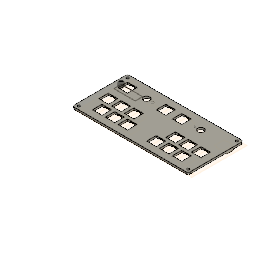
Keyboard Plate (Autodesk Fusion 360 design; units mm, degrees)
Autodesk Fusion 360 part; units mm, degrees
(part 1 of 2)
sketch "fe59f99c189e2fed6147eb83aa4c487c15dc8bc6_switch" plane through (0, 0, 0) normal (0, 0, 1) x (1, 0, 0)
  line L0 (34.1437, 24.5994) -> (34.1437, 10.5999)
  line L1 (110.63, 43.6492) -> (124.631, 43.6492)
  line L2 (58.2429, 24.5994) -> (72.2422, 24.5994)
  line L3 (110.63, 29.6499) -> (110.63, 43.6492)
  line L4 (29.6692, 43.6492) -> (43.6686, 43.6492)
  line L5 (43.6686, 29.6499) -> (29.6692, 29.6499)
  line L6 (124.631, 29.6499) -> (110.63, 29.6499)
  line L7 (101.105, 10.5999) -> (101.105, 24.5994)
  line L8 (120.155, 24.5994) -> (134.156, 24.5994)
  line L9 (53.1922, 24.5994) -> (53.1922, 10.5999)
  line L10 (129.68, 29.6499) -> (129.68, 43.6492)
  line L11 (67.7693, 72.2256) -> (81.7686, 72.2256)
  line L12 (148.73, 43.6492) -> (162.731, 43.6492)
  line L13 (115.106, 10.5999) -> (101.105, 10.5999)
  line L14 (20.1428, 10.5999) -> (20.1428, 24.5994)
  line L15 (148.73, 29.6499) -> (148.73, 43.6492)
  line L16 (34.1437, 10.5999) -> (20.1428, 10.5999)
  line L17 (62.7186, 43.6492) -> (62.7186, 29.6499)
  line L18 (24.6187, 29.6499) -> (10.6178, 29.6499)
  line L19 (120.155, 10.5999) -> (120.155, 24.5994)
  line L20 (134.156, 24.5994) -> (134.156, 10.5999)
  line L21 (153.206, 10.5999) -> (139.205, 10.5999)
  line L22 (10.6178, 43.6492) -> (24.6187, 43.6492)
  line L23 (143.681, 43.6492) -> (143.681, 29.6499)
  line L24 (139.205, 24.5994) -> (153.206, 24.5994)
  line L25 (20.1428, 24.5994) -> (34.1437, 24.5994)
  line L26 (39.1929, 10.5999) -> (39.1929, 24.5994)
  line L27 (162.731, 29.6499) -> (148.73, 29.6499)
  line L28 (124.631, 43.6492) -> (124.631, 29.6499)
  line L29 (58.2429, 10.5999) -> (58.2429, 24.5994)
  line L30 (134.156, 10.5999) -> (120.155, 10.5999)
  line L31 (48.7193, 43.6492) -> (62.7186, 43.6492)
  line L32 (153.206, 24.5994) -> (153.206, 10.5999)
  line L33 (143.681, 29.6499) -> (129.68, 29.6499)
  line L34 (162.731, 58.2249) -> (148.73, 58.2249)
  line L35 (115.106, 24.5994) -> (115.106, 10.5999)
  line L36 (0.0937, 82.7497) -> (173.257, 82.7497)
  line L37 (53.1922, 10.5999) -> (39.1929, 10.5999)
  line L38 (10.6178, 29.6499) -> (10.6178, 43.6492)
  line L39 (43.6686, 43.6492) -> (43.6686, 29.6499)
  line L40 (105.581, 58.2249) -> (91.5804, 58.2249)
  line L41 (67.7693, 58.2249) -> (67.7693, 72.2256)
  line L42 (62.7186, 29.6499) -> (48.7193, 29.6499)
  line L43 (81.7686, 58.2249) -> (67.7693, 58.2249)
  line L44 (148.73, 72.2256) -> (162.731, 72.2256)
  line L45 (0.0937, 0.0744) -> (0.0937, 82.7497)
  line L46 (173.257, 0.0744) -> (0.0937, 0.0744)
  line L47 (72.2422, 10.5999) -> (58.2429, 10.5999)
  line L48 (39.1929, 24.5994) -> (53.1922, 24.5994)
  line L49 (173.257, 82.7497) -> (173.257, 0.0744)
  line L50 (72.2422, 24.5994) -> (72.2422, 10.5999)
  line L51 (29.6692, 29.6499) -> (29.6692, 43.6492)
  line L52 (148.73, 58.2249) -> (148.73, 72.2256)
  line L53 (162.731, 43.6492) -> (162.731, 29.6499)
  line L54 (91.5804, 72.2256) -> (105.581, 72.2256)
  line L55 (139.205, 10.5999) -> (139.205, 24.5994)
  line L56 (91.5804, 58.2249) -> (91.5804, 72.2256)
  line L57 (81.7686, 72.2256) -> (81.7686, 58.2249)
  line L58 (24.6187, 43.6492) -> (24.6187, 29.6499)
  line L59 (48.7193, 29.6499) -> (48.7193, 43.6492)
  line L60 (129.68, 43.6492) -> (143.681, 43.6492)
  line L61 (162.731, 72.2256) -> (162.731, 58.2249)
  line L62 (105.581, 72.2256) -> (105.581, 58.2249)
  line L63 (101.105, 24.5994) -> (115.106, 24.5994)
extrude "Extrude1" add sketch "fe59f99c189e2fed6147eb83aa4c487c15dc8bc6_switch" along normal blind 3
sketch "Sketch2" plane through (0, 0, 3) normal (0, 0, 1) x (-1, 0, 0)
  line L0 (-39.1929, -10.5999) -> (-39.1929, -24.5994)
  line L1 (-39.1929, -24.5994) -> (-53.1922, -24.5994)
  line L2 (-53.1922, -24.5994) -> (-53.1922, -10.5999)
  line L3 (-53.1922, -10.5999) -> (-39.1929, -10.5999)
  line L4 (-110.63, -43.6492) -> (-124.631, -43.6492)
  line L5 (-124.631, -43.6492) -> (-124.631, -29.6499)
  line L6 (-124.631, -29.6499) -> (-110.63, -29.6499)
  line L7 (-110.63, -29.6499) -> (-110.63, -43.6492)
  line L8 (-134.156, -24.5994) -> (-134.156, -10.5999)
  line L9 (-134.156, -10.5999) -> (-120.155, -10.5999)
  line L10 (-120.155, -10.5999) -> (-120.155, -24.5994)
  line L11 (-120.155, -24.5994) -> (-134.156, -24.5994)
  line L12 (-20.1428, -10.5999) -> (-20.1428, -24.5994)
  line L13 (-20.1428, -24.5994) -> (-34.1437, -24.5994)
  line L14 (-34.1437, -24.5994) -> (-34.1437, -10.5999)
  line L15 (-34.1437, -10.5999) -> (-20.1428, -10.5999)
  line L16 (-148.73, -43.6492) -> (-162.731, -43.6492)
  line L17 (-162.731, -43.6492) -> (-162.731, -29.6499)
  line L18 (-162.731, -29.6499) -> (-148.73, -29.6499)
  line L19 (-148.73, -29.6499) -> (-148.73, -43.6492)
  line L20 (-58.2429, -24.5994) -> (-72.2422, -24.5994)
  line L21 (-72.2422, -24.5994) -> (-72.2422, -10.5999)
  line L22 (-72.2422, -10.5999) -> (-58.2429, -10.5999)
  line L23 (-58.2429, -10.5999) -> (-58.2429, -24.5994)
  line L24 (-43.6686, -29.6499) -> (-29.6692, -29.6499)
  line L25 (-29.6692, -29.6499) -> (-29.6692, -43.6492)
  line L26 (-29.6692, -43.6492) -> (-43.6686, -43.6492)
  line L27 (-43.6686, -43.6492) -> (-43.6686, -29.6499)
  line L28 (-153.206, -10.5999) -> (-139.205, -10.5999)
  line L29 (-139.205, -10.5999) -> (-139.205, -24.5994)
  line L30 (-139.205, -24.5994) -> (-153.206, -24.5994)
  line L31 (-153.206, -24.5994) -> (-153.206, -10.5999)
  line L32 (-10.6178, -43.6492) -> (-24.6187, -43.6492)
  line L33 (-24.6187, -43.6492) -> (-24.6187, -29.6499)
  line L34 (-24.6187, -29.6499) -> (-10.6178, -29.6499)
  line L35 (-10.6178, -29.6499) -> (-10.6178, -43.6492)
  line L36 (-62.7186, -29.6499) -> (-48.7193, -29.6499)
  line L37 (-48.7193, -29.6499) -> (-48.7193, -43.6492)
  line L38 (-48.7193, -43.6492) -> (-62.7186, -43.6492)
  line L39 (-62.7186, -43.6492) -> (-62.7186, -29.6499)
  line L40 (-67.7693, -72.2256) -> (-81.7686, -72.2256)
  line L41 (-81.7686, -72.2256) -> (-81.7686, -58.2249)
  line L42 (-81.7686, -58.2249) -> (-67.7693, -58.2249)
  line L43 (-67.7693, -58.2249) -> (-67.7693, -72.2256)
  line L44 (-129.68, -29.6499) -> (-129.68, -43.6492)
  line L45 (-129.68, -43.6492) -> (-143.681, -43.6492)
  line L46 (-143.681, -43.6492) -> (-143.681, -29.6499)
  line L47 (-143.681, -29.6499) -> (-129.68, -29.6499)
  line L48 (-148.73, -72.2256) -> (-162.731, -72.2256)
  line L49 (-162.731, -72.2256) -> (-162.731, -58.2249)
  line L50 (-162.731, -58.2249) -> (-148.73, -58.2249)
  line L51 (-148.73, -58.2249) -> (-148.73, -72.2256)
  line L52 (-101.105, -10.5999) -> (-101.105, -24.5994)
  line L53 (-101.105, -24.5994) -> (-115.106, -24.5994)
  line L54 (-115.106, -24.5994) -> (-115.106, -10.5999)
  line L55 (-115.106, -10.5999) -> (-101.105, -10.5999)
  line L56 (-91.5804, -72.2256) -> (-105.581, -72.2256)
  line L57 (-105.581, -72.2256) -> (-105.581, -58.2249)
  line L58 (-105.581, -58.2249) -> (-91.5804, -58.2249)
  line L59 (-91.5804, -58.2249) -> (-91.5804, -72.2256)
  line L60 (-173.257, -82.7497) -> (-0.0937, -82.7497)
  line L61 (-0.0937, -82.7497) -> (-0.0937, -0.0744)
  line L62 (-0.0937, -0.0744) -> (-173.257, -0.0744)
  line L63 (-173.257, -0.0744) -> (-173.257, -82.7497)
  line L64 (-71.769, -72.2256) -> (-77.769, -72.2256)
  line L65 (-77.769, -72.2256) -> (-77.769, -73.2256)
  line L66 (-77.769, -73.2256) -> (-71.769, -73.2256)
  line L67 (-71.769, -73.2256) -> (-71.769, -72.2256)
  line L68 (-71.769, -58.2249) -> (-77.769, -58.2249)
  line L69 (-77.769, -58.2249) -> (-77.769, -57.2249)
  line L70 (-77.769, -57.2249) -> (-71.769, -57.2249)
  line L71 (-71.769, -57.2249) -> (-71.769, -58.2249)
  line L72 (-95.5807, -58.2249) -> (-101.5807, -58.2249)
  line L73 (-101.5807, -73.2256) -> (-95.5807, -73.2256)
  line L74 (-101.5807, -72.2256) -> (-101.5807, -73.2256)
  line L75 (-95.5807, -72.2256) -> (-101.5807, -72.2256)
  line L76 (-95.5807, -73.2256) -> (-95.5807, -72.2256)
  line L77 (-101.5807, -58.2249) -> (-101.5807, -57.2249)
  line L78 (-95.5807, -57.2249) -> (-95.5807, -58.2249)
  line L79 (-101.5807, -57.2249) -> (-95.5807, -57.2249)
  line L80 (-152.7305, -58.2249) -> (-158.7305, -58.2249)
  line L81 (-158.7305, -73.2256) -> (-152.7305, -73.2256)
  line L82 (-158.7305, -72.2256) -> (-158.7305, -73.2256)
  line L83 (-152.7305, -72.2256) -> (-158.7305, -72.2256)
  line L84 (-152.7305, -73.2256) -> (-152.7305, -72.2256)
  line L85 (-158.7305, -58.2249) -> (-158.7305, -57.2249)
  line L86 (-152.7305, -57.2249) -> (-152.7305, -58.2249)
  line L87 (-158.7305, -57.2249) -> (-152.7305, -57.2249)
  line L88 (-14.6183, -43.6492) -> (-20.6183, -43.6492)
  line L89 (-20.6183, -43.6492) -> (-20.6183, -44.6492)
  line L90 (-20.6183, -44.6492) -> (-14.6183, -44.6492)
  line L91 (-14.6183, -44.6492) -> (-14.6183, -43.6492)
  line L92 (-14.6183, -29.6499) -> (-20.6183, -29.6499)
  line L93 (-20.6183, -29.6499) -> (-20.6183, -28.6499)
  line L94 (-20.6183, -28.6499) -> (-14.6183, -28.6499)
  line L95 (-14.6183, -28.6499) -> (-14.6183, -29.6499)
  line L96 (-58.719, -29.6499) -> (-58.719, -28.6499)
  line L97 (-58.719, -28.6499) -> (-52.7189, -28.6499)
  line L98 (-58.7189, -44.6492) -> (-52.7189, -44.6492)
  line L99 (-52.7189, -29.6499) -> (-58.719, -29.6499)
  line L100 (-52.7189, -43.6492) -> (-58.7189, -43.6492)
  line L101 (-52.7189, -44.6492) -> (-52.7189, -43.6492)
  line L102 (-58.7189, -43.6492) -> (-58.7189, -44.6492)
  line L103 (-52.7189, -28.6499) -> (-52.7189, -29.6499)
  line L104 (-39.6689, -29.6499) -> (-39.6689, -28.6499)
  line L105 (-39.6689, -28.6499) -> (-33.6689, -28.6499)
  line L106 (-39.6689, -44.6492) -> (-33.6689, -44.6492)
  line L107 (-33.6689, -29.6499) -> (-39.6689, -29.6499)
  line L108 (-33.6689, -43.6492) -> (-39.6689, -43.6492)
  line L109 (-33.6689, -44.6492) -> (-33.6689, -43.6492)
  line L110 (-39.6689, -43.6492) -> (-39.6689, -44.6492)
  line L111 (-33.6689, -28.6499) -> (-33.6689, -29.6499)
  line L112 (-120.6305, -29.6499) -> (-120.6305, -28.6499)
  line L113 (-120.6305, -28.6499) -> (-114.6305, -28.6499)
  line L114 (-120.6305, -44.6492) -> (-114.6305, -44.6492)
  line L115 (-114.6305, -29.6499) -> (-120.6305, -29.6499)
  line L116 (-114.6305, -43.6492) -> (-120.6305, -43.6492)
  line L117 (-114.6305, -44.6492) -> (-114.6305, -43.6492)
  line L118 (-120.6305, -43.6492) -> (-120.6305, -44.6492)
  line L119 (-114.6305, -28.6499) -> (-114.6305, -29.6499)
  line L120 (-139.6805, -29.6499) -> (-139.6805, -28.6499)
  line L121 (-139.6805, -28.6499) -> (-133.6805, -28.6499)
  line L122 (-139.6805, -44.6492) -> (-133.6805, -44.6492)
  line L123 (-133.6805, -29.6499) -> (-139.6805, -29.6499)
  line L124 (-133.6805, -43.6492) -> (-139.6805, -43.6492)
  line L125 (-133.6805, -44.6492) -> (-133.6805, -43.6492)
  line L126 (-139.6805, -43.6492) -> (-139.6805, -44.6492)
  line L127 (-133.6805, -28.6499) -> (-133.6805, -29.6499)
  line L128 (-158.7305, -29.6499) -> (-158.7305, -28.6499)
  line L129 (-158.7305, -28.6499) -> (-152.7305, -28.6499)
  line L130 (-158.7305, -44.6492) -> (-152.7305, -44.6492)
  line L131 (-152.7305, -29.6499) -> (-158.7305, -29.6499)
  line L132 (-152.7305, -43.6492) -> (-158.7305, -43.6492)
  line L133 (-152.7305, -44.6492) -> (-152.7305, -43.6492)
  line L134 (-158.7305, -43.6492) -> (-158.7305, -44.6492)
  line L135 (-152.7305, -28.6499) -> (-152.7305, -29.6499)
  line L136 (-24.1433, -24.5994) -> (-30.1433, -24.5994)
  line L137 (-30.1433, -24.5994) -> (-30.1433, -25.5994)
  line L138 (-30.1433, -25.5994) -> (-24.1433, -25.5994)
  line L139 (-24.1433, -25.5994) -> (-24.1433, -24.5994)
  line L140 (-24.1433, -10.5999) -> (-30.1433, -10.5999)
  line L141 (-30.1433, -10.5999) -> (-30.1433, -9.5999)
  line L142 (-30.1433, -9.5999) -> (-24.1433, -9.5999)
  line L143 (-24.1433, -9.5999) -> (-24.1433, -10.5999)
  line L144 (-43.1926, -9.5999) -> (-43.1926, -10.5999)
  line L145 (-49.1926, -9.5999) -> (-43.1926, -9.5999)
  line L146 (-49.1926, -24.5994) -> (-49.1926, -25.5994)
  line L147 (-43.1926, -10.5999) -> (-49.1926, -10.5999)
  line L148 (-43.1926, -24.5994) -> (-49.1926, -24.5994)
  line L149 (-43.1926, -25.5994) -> (-43.1926, -24.5994)
  line L150 (-49.1926, -10.5999) -> (-49.1926, -9.5999)
  line L151 (-49.1926, -25.5994) -> (-43.1926, -25.5994)
  line L152 (-62.2426, -9.5999) -> (-62.2426, -10.5999)
  line L153 (-68.2426, -9.5999) -> (-62.2426, -9.5999)
  line L154 (-68.2425, -24.5994) -> (-68.2425, -25.5994)
  line L155 (-62.2426, -10.5999) -> (-68.2426, -10.5999)
  line L156 (-62.2426, -24.5994) -> (-68.2425, -24.5994)
  line L157 (-62.2426, -25.5994) -> (-62.2426, -24.5994)
  line L158 (-68.2426, -10.5999) -> (-68.2426, -9.5999)
  line L159 (-68.2425, -25.5994) -> (-62.2425, -25.5994)
  line L160 (-105.1055, -9.5999) -> (-105.1055, -10.5999)
  line L161 (-111.1055, -9.5999) -> (-105.1055, -9.5999)
  line L162 (-111.1055, -24.5994) -> (-111.1055, -25.5994)
  line L163 (-105.1055, -10.5999) -> (-111.1055, -10.5999)
  line L164 (-105.1055, -24.5994) -> (-111.1055, -24.5994)
  line L165 (-105.1055, -25.5994) -> (-105.1055, -24.5994)
  line L166 (-111.1055, -10.5999) -> (-111.1055, -9.5999)
  line L167 (-111.1055, -25.5994) -> (-105.1055, -25.5994)
  line L168 (-124.1555, -9.5999) -> (-124.1555, -10.5999)
  line L169 (-130.1555, -9.5999) -> (-124.1555, -9.5999)
  line L170 (-130.1555, -24.5994) -> (-130.1555, -25.5994)
  line L171 (-124.1555, -10.5999) -> (-130.1555, -10.5999)
  line L172 (-124.1555, -24.5994) -> (-130.1555, -24.5994)
  line L173 (-124.1555, -25.5994) -> (-124.1555, -24.5994)
  line L174 (-130.1555, -10.5999) -> (-130.1555, -9.5999)
  line L175 (-130.1555, -25.5994) -> (-124.1555, -25.5994)
  line L176 (-143.2055, -9.5999) -> (-143.2055, -10.5999)
  line L177 (-149.2055, -9.5999) -> (-143.2055, -9.5999)
  line L178 (-149.2055, -24.5994) -> (-149.2055, -25.5994)
  line L179 (-143.2055, -10.5999) -> (-149.2055, -10.5999)
  line L180 (-143.2055, -24.5994) -> (-149.2055, -24.5994)
  line L181 (-143.2055, -25.5994) -> (-143.2055, -24.5994)
  line L182 (-149.2055, -10.5999) -> (-149.2055, -9.5999)
  line L183 (-149.2055, -25.5994) -> (-143.2055, -25.5994)
  dimension "d3" = 6
  dimension "d4" = 1
  dimension "d5" = 6
  dimension "d6" = 1
  dimension "d7" = 6
  dimension "d8" = 1
  dimension "d9" = 6
  dimension "d10" = 1
  dimension "d11" = 6
  dimension "d12" = 1
  dimension "d13" = 6
  dimension "d14" = 1
  dimension "d15" = 6
  dimension "d16" = 1
  dimension "d17" = 6
  dimension "d18" = 1
  dimension "d19" = 6
  dimension "d20" = 1
  dimension "d21" = 6
  dimension "d22" = 1
  dimension "d23" = 6
  dimension "d24" = 1
  dimension "d25" = 6
  dimension "d26" = 1
  dimension "d27" = 6
  dimension "d28" = 1
  dimension "d29" = 6
  dimension "d30" = 1
  dimension "d31" = 6
  dimension "d32" = 1
  dimension "d33" = 6
  dimension "d34" = 1
  dimension "d35" = 6
  dimension "d36" = 1
  dimension "d37" = 6
  dimension "d38" = 1
  dimension "d39" = 6
  dimension "d40" = 1
  dimension "d41" = 6
  dimension "d42" = 1
  dimension "d43" = 6
  dimension "d44" = 1
  dimension "d45" = 6
  dimension "d46" = 1
  dimension "d47" = 6
  dimension "d48" = 1
  dimension "d49" = 6
  dimension "d50" = 1
  dimension "d51" = 6
  dimension "d52" = 1
  dimension "d53" = 6
  dimension "d54" = 1
  dimension "d55" = 6
  dimension "d56" = 1
  dimension "d57" = 6
  dimension "d58" = 1
  dimension "d59" = 6
  dimension "d60" = 1
  dimension "d61" = 6
  dimension "d62" = 1
  constraint horizontal L64
  constraint vertical L65
  constraint horizontal L66
  constraint vertical L67
  constraint coincident L40 L64.start
  constraint horizontal L68
  constraint vertical L69
  constraint horizontal L70
  constraint vertical L71
  constraint coincident L42 L68.start
  constraint horizontal L75
  constraint vertical L74
  constraint horizontal L73
  constraint vertical L76
  constraint horizontal L72
  constraint vertical L77
  constraint horizontal L79
  constraint vertical L78
  constraint horizontal L83
  constraint vertical L82
  constraint horizontal L81
  constraint vertical L84
  constraint horizontal L80
  constraint vertical L85
  constraint horizontal L87
  constraint vertical L86
  constraint horizontal L88
  constraint vertical L89
  constraint horizontal L90
  constraint vertical L91
  constraint coincident L32 L88.start
  constraint horizontal L92
  constraint vertical L93
  constraint horizontal L94
  constraint vertical L95
  constraint coincident L34 L92.start
  constraint horizontal L100
  constraint vertical L102
  constraint horizontal L98
  constraint vertical L101
  constraint horizontal L99
  constraint vertical L96
  constraint horizontal L97
  constraint vertical L103
  constraint horizontal L108
  constraint vertical L110
  constraint horizontal L106
  constraint vertical L109
  constraint horizontal L107
  constraint vertical L104
  constraint horizontal L105
  constraint vertical L111
  constraint horizontal L116
  constraint vertical L118
  constraint horizontal L114
  constraint vertical L117
  constraint horizontal L115
  constraint vertical L112
  constraint horizontal L113
  constraint vertical L119
  constraint horizontal L124
  constraint vertical L126
  constraint horizontal L122
  constraint vertical L125
  constraint horizontal L123
  constraint vertical L120
  constraint horizontal L121
  constraint vertical L127
  constraint horizontal L132
  constraint vertical L134
  constraint horizontal L130
  constraint vertical L133
  constraint horizontal L131
  constraint vertical L128
  constraint horizontal L129
  constraint vertical L135
  constraint horizontal L136
  constraint vertical L137
  constraint horizontal L138
  constraint vertical L139
  constraint coincident L13 L136.start
  constraint horizontal L140
  constraint vertical L141
  constraint horizontal L142
  constraint vertical L143
  constraint coincident L15 L140.start
  constraint horizontal L148
  constraint vertical L146
  constraint horizontal L151
  constraint vertical L149
  constraint horizontal L147
  constraint vertical L150
  constraint horizontal L145
  constraint vertical L144
  constraint horizontal L156
  constraint vertical L154
  constraint horizontal L159
  constraint vertical L157
  constraint horizontal L155
  constraint vertical L158
  constraint horizontal L153
  constraint vertical L152
  constraint horizontal L164
  constraint vertical L162
  constraint horizontal L167
  constraint vertical L165
  constraint horizontal L163
  constraint vertical L166
  constraint horizontal L161
  constraint vertical L160
  constraint horizontal L172
  constraint vertical L170
  constraint horizontal L175
  constraint vertical L173
  constraint horizontal L171
  constraint vertical L174
  constraint horizontal L169
  constraint vertical L168
  constraint horizontal L180
  constraint vertical L178
  constraint horizontal L183
  constraint vertical L181
  constraint horizontal L179
  constraint vertical L182
  constraint horizontal L177
  constraint vertical L176
  constraint midpoint L40 L64
  constraint midpoint L56 L75
  constraint midpoint L58 L72
  constraint midpoint L42 L68
  constraint midpoint L48 L83
  constraint midpoint L50 L80
  constraint midpoint L16 L132
  constraint midpoint L45 L124
  constraint midpoint L18 L131
  constraint midpoint L47 L123
  constraint midpoint L6 L115
  constraint midpoint L4 L116
  constraint midpoint L38 L100
  constraint midpoint L36 L99
  constraint midpoint L24 L107
  constraint midpoint L26 L108
  constraint midpoint L32 L88
  constraint midpoint L34 L92
  constraint midpoint L13 L136
  constraint midpoint L15 L140
  constraint midpoint L3 L147
  constraint midpoint L1 L148
  constraint midpoint L20 L156
  constraint midpoint L22 L155
  constraint midpoint L55 L163
  constraint midpoint L53 L164
  constraint midpoint L11 L172
  constraint midpoint L9 L171
  constraint midpoint L28 L179
  constraint midpoint L30 L180
  measures "d3" distance of L64.start L64.end
  measures "d4" distance of L64.start L66.end
  measures "d5" distance of L68.start L68.end
  measures "d6" distance of L68.start L70.end
  measures "d7" distance of L75.start L74.start
  measures "d8" distance of L75.start L73.end
  measures "d9" distance of L72.start L72.end
  measures "d10" distance of L72.start L78.start
  measures "d11" distance of L83.start L82.start
  measures "d12" distance of L83.start L81.end
  measures "d13" distance of L80.start L80.end
  measures "d14" distance of L80.start L86.start
  measures "d15" distance of L88.start L88.end
  measures "d16" distance of L88.start L90.end
  measures "d17" distance of L92.start L92.end
  measures "d18" distance of L92.start L94.end
  measures "d19" distance of L100.end L100.start
  measures "d20" distance of L100.start L98.end
  measures "d21" distance of L96.start L99.start
  measures "d22" distance of L97.end L99.start
  measures "d23" distance of L108.end L108.start
  measures "d24" distance of L108.start L106.end
  measures "d25" distance of L104.start L107.start
  measures "d26" distance of L105.end L107.start
  measures "d27" distance of L116.end L116.start
  measures "d28" distance of L116.start L114.end
  measures "d29" distance of L112.start L115.start
  measures "d30" distance of L113.end L115.start
  measures "d31" distance of L124.end L124.start
  measures "d32" distance of L124.start L122.end
  measures "d33" distance of L120.start L123.start
  measures "d34" distance of L121.end L123.start
  measures "d35" distance of L132.end L132.start
  measures "d36" distance of L132.start L130.end
  measures "d37" distance of L128.start L131.start
  measures "d38" distance of L129.end L131.start
  measures "d39" distance of L136.start L136.end
  measures "d40" distance of L136.start L138.end
  measures "d41" distance of L140.start L140.end
  measures "d42" distance of L140.start L142.end
  measures "d43" distance of L148.start L146.start
  measures "d44" distance of L149.start L148.start
  measures "d45" distance of L144.end L147.end
  measures "d46" distance of L144.start L144.end
  measures "d47" distance of L156.start L154.start
  measures "d48" distance of L157.start L156.start
  measures "d49" distance of L152.end L155.end
  measures "d50" distance of L152.start L152.end
  measures "d51" distance of L164.start L162.start
  measures "d52" distance of L165.start L164.start
  measures "d53" distance of L160.end L163.end
  measures "d54" distance of L160.start L160.end
  measures "d55" distance of L172.start L170.start
  measures "d56" distance of L173.start L172.start
  measures "d57" distance of L168.end L171.end
  measures "d58" distance of L168.start L168.end
  measures "d59" distance of L180.start L178.start
  measures "d60" distance of L181.start L180.start
  measures "d61" distance of L176.end L179.end
  measures "d62" distance of L176.start L176.end
extrude "Extrude2" cut sketch "Sketch2" against normal blind 1.5 contours L3 L144 L145 L147 L150 | L1 L146 L148 L149 L151 | L4 L114 L116 L117 L118 | L6 L112 L113 L115 L119 | L11 L170 L172 L173 L175 | L9 L168 L169 L171 L174 | L15 L140 L141 L142 L143 | L13 L136 L137 L138 L139 | L16 L130 L132 L133 L134 | L18 L128 L129 L131 L135 | L20 L154 L156 L157 L159 | L22 L152 L153 L155 L158 | L24 L104 L105 L107 L111 | L26 L106 L108 L109 L110 | L28 L176 L177 L179 L182 | L30 L178 L180 L181 L183 | L32 L88 L89 L90 L91 | L34 L92 L93 L94 L95 | L36 L96 L97 L99 L103 | L38 L98 L100 L101 L102 | L40 L64 L65 L66 L67 | L42 L68 L69 L70 L71 | L47 L120 L121 L123 L127 | L45 L122 L124 L125 L126 | L48 L81 L82 L83 L84 | L50 L80 L85 L86 L87 | L55 L160 L161 L163 L166 | L53 L162 L164 L165 L167 | L56 L73 L74 L75 L76 | L58 L72 L77 L78 L79
sketch "Sketch3" plane through (0, 0, 3) normal (0, 0, 1) x (-1, 0, 0)
  line L0 (-173.257, -82.7497) -> (-0.0937, -82.7497)
  line L1 (-0.0937, -82.7497) -> (-0.0937, -0.0744)
  line L2 (-0.0937, -0.0744) -> (-173.257, -0.0744)
  line L3 (-173.257, -0.0744) -> (-173.257, -82.7497)
  line L4 (-101.5807, -58.2249) -> (-101.5807, -57.2249)
  line L5 (-101.5807, -57.2249) -> (-95.5807, -57.2249)
  line L6 (-95.5807, -57.2249) -> (-95.5807, -58.2249)
  line L7 (-95.5807, -58.2249) -> (-91.5804, -58.2249)
  line L8 (-91.5804, -58.2249) -> (-91.5804, -72.2256)
  line L9 (-91.5804, -72.2256) -> (-95.5807, -72.2256)
  line L10 (-95.5807, -72.2256) -> (-95.5807, -73.2256)
  line L11 (-95.5807, -73.2256) -> (-101.5807, -73.2256)
  line L12 (-101.5807, -73.2256) -> (-101.5807, -72.2256)
  line L13 (-101.5807, -72.2256) -> (-105.581, -72.2256)
  line L14 (-105.581, -72.2256) -> (-105.581, -58.2249)
  line L15 (-105.581, -58.2249) -> (-101.5807, -58.2249)
  line L16 (-152.7305, -72.2256) -> (-152.7305, -73.2256)
  line L17 (-152.7305, -73.2256) -> (-158.7305, -73.2256)
  line L18 (-158.7305, -73.2256) -> (-158.7305, -72.2256)
  line L19 (-158.7305, -72.2256) -> (-162.731, -72.2256)
  line L20 (-162.731, -72.2256) -> (-162.731, -58.2249)
  line L21 (-162.731, -58.2249) -> (-158.7305, -58.2249)
  line L22 (-158.7305, -58.2249) -> (-158.7305, -57.2249)
  line L23 (-158.7305, -57.2249) -> (-152.7305, -57.2249)
  line L24 (-152.7305, -57.2249) -> (-152.7305, -58.2249)
  line L25 (-152.7305, -58.2249) -> (-148.73, -58.2249)
  line L26 (-148.73, -58.2249) -> (-148.73, -72.2256)
  line L27 (-148.73, -72.2256) -> (-152.7305, -72.2256)
  line L28 (-58.7189, -44.6492) -> (-58.7189, -43.6492)
  line L29 (-58.7189, -43.6492) -> (-62.7186, -43.6492)
  line L30 (-62.7186, -43.6492) -> (-62.7186, -29.6499)
  line L31 (-62.7186, -29.6499) -> (-58.719, -29.6499)
  line L32 (-58.719, -29.6499) -> (-58.719, -28.6499)
  line L33 (-58.719, -28.6499) -> (-52.7189, -28.6499)
  line L34 (-52.7189, -28.6499) -> (-52.7189, -29.6499)
  line L35 (-52.7189, -29.6499) -> (-48.7193, -29.6499)
  line L36 (-48.7193, -29.6499) -> (-48.7193, -43.6492)
  line L37 (-48.7193, -43.6492) -> (-52.7189, -43.6492)
  line L38 (-52.7189, -43.6492) -> (-52.7189, -44.6492)
  line L39 (-52.7189, -44.6492) -> (-58.7189, -44.6492)
  line L40 (-24.1433, -24.5994) -> (-24.1433, -25.5994)
  line L41 (-24.1433, -25.5994) -> (-30.1433, -25.5994)
  line L42 (-30.1433, -25.5994) -> (-30.1433, -24.5994)
  line L43 (-30.1433, -24.5994) -> (-34.1437, -24.5994)
  line L44 (-34.1437, -24.5994) -> (-34.1437, -10.5999)
  line L45 (-34.1437, -10.5999) -> (-30.1433, -10.5999)
  line L46 (-30.1433, -10.5999) -> (-30.1433, -9.5999)
  line L47 (-30.1433, -9.5999) -> (-24.1433, -9.5999)
  line L48 (-24.1433, -9.5999) -> (-24.1433, -10.5999)
  line L49 (-24.1433, -10.5999) -> (-20.1428, -10.5999)
  line L50 (-20.1428, -10.5999) -> (-20.1428, -24.5994)
  line L51 (-20.1428, -24.5994) -> (-24.1433, -24.5994)
  line L52 (-71.769, -72.2256) -> (-71.769, -73.2256)
  line L53 (-71.769, -73.2256) -> (-77.769, -73.2256)
  line L54 (-77.769, -73.2256) -> (-77.769, -72.2256)
  line L55 (-77.769, -72.2256) -> (-81.7686, -72.2256)
  line L56 (-81.7686, -72.2256) -> (-81.7686, -58.2249)
  line L57 (-81.7686, -58.2249) -> (-77.769, -58.2249)
  line L58 (-77.769, -58.2249) -> (-77.769, -57.2249)
  line L59 (-77.769, -57.2249) -> (-71.769, -57.2249)
  line L60 (-71.769, -57.2249) -> (-71.769, -58.2249)
  line L61 (-71.769, -58.2249) -> (-67.7693, -58.2249)
  line L62 (-67.7693, -58.2249) -> (-67.7693, -72.2256)
  line L63 (-67.7693, -72.2256) -> (-71.769, -72.2256)
  line L64 (-158.7305, -44.6492) -> (-158.7305, -43.6492)
  line L65 (-158.7305, -43.6492) -> (-162.731, -43.6492)
  line L66 (-162.731, -43.6492) -> (-162.731, -29.6499)
  line L67 (-162.731, -29.6499) -> (-158.7305, -29.6499)
  line L68 (-158.7305, -29.6499) -> (-158.7305, -28.6499)
  line L69 (-158.7305, -28.6499) -> (-152.7305, -28.6499)
  line L70 (-152.7305, -28.6499) -> (-152.7305, -29.6499)
  line L71 (-152.7305, -29.6499) -> (-148.73, -29.6499)
  line L72 (-148.73, -29.6499) -> (-148.73, -43.6492)
  line L73 (-148.73, -43.6492) -> (-152.7305, -43.6492)
  line L74 (-152.7305, -43.6492) -> (-152.7305, -44.6492)
  line L75 (-152.7305, -44.6492) -> (-158.7305, -44.6492)
  line L76 (-149.2055, -25.5994) -> (-149.2055, -24.5994)
  line L77 (-149.2055, -24.5994) -> (-153.206, -24.5994)
  line L78 (-153.206, -24.5994) -> (-153.206, -10.5999)
  line L79 (-153.206, -10.5999) -> (-149.2055, -10.5999)
  line L80 (-149.2055, -10.5999) -> (-149.2055, -9.5999)
  line L81 (-149.2055, -9.5999) -> (-143.2055, -9.5999)
  line L82 (-143.2055, -9.5999) -> (-143.2055, -10.5999)
  line L83 (-143.2055, -10.5999) -> (-139.205, -10.5999)
  line L84 (-139.205, -10.5999) -> (-139.205, -24.5994)
  line L85 (-139.205, -24.5994) -> (-143.2055, -24.5994)
  line L86 (-143.2055, -24.5994) -> (-143.2055, -25.5994)
  line L87 (-143.2055, -25.5994) -> (-149.2055, -25.5994)
  line L88 (-62.2426, -9.5999) -> (-62.2426, -10.5999)
  line L89 (-62.2426, -10.5999) -> (-58.2429, -10.5999)
  line L90 (-58.2429, -10.5999) -> (-58.2429, -24.5994)
  line L91 (-58.2429, -24.5994) -> (-62.2426, -24.5994)
  line L92 (-62.2426, -24.5994) -> (-62.2426, -25.5994)
  line L93 (-62.2426, -25.5994) -> (-68.2425, -25.5994)
  line L94 (-68.2425, -25.5994) -> (-68.2425, -24.5994)
  line L95 (-68.2425, -24.5994) -> (-72.2422, -24.5994)
  line L96 (-72.2422, -24.5994) -> (-72.2422, -10.5999)
  line L97 (-72.2422, -10.5999) -> (-68.2426, -10.5999)
  line L98 (-68.2426, -10.5999) -> (-68.2426, -9.5999)
  line L99 (-68.2426, -9.5999) -> (-62.2426, -9.5999)
  line L100 (-114.6305, -28.6499) -> (-114.6305, -29.6499)
  line L101 (-114.6305, -29.6499) -> (-110.63, -29.6499)
  line L102 (-110.63, -29.6499) -> (-110.63, -43.6492)
  line L103 (-110.63, -43.6492) -> (-114.6305, -43.6492)
  line L104 (-114.6305, -43.6492) -> (-114.6305, -44.6492)
  line L105 (-114.6305, -44.6492) -> (-120.6305, -44.6492)
  line L106 (-120.6305, -44.6492) -> (-120.6305, -43.6492)
  line L107 (-120.6305, -43.6492) -> (-124.631, -43.6492)
  line L108 (-124.631, -43.6492) -> (-124.631, -29.6499)
  line L109 (-124.631, -29.6499) -> (-120.6305, -29.6499)
  line L110 (-120.6305, -29.6499) -> (-120.6305, -28.6499)
  line L111 (-120.6305, -28.6499) -> (-114.6305, -28.6499)
  line L112 (-111.1055, -25.5994) -> (-111.1055, -24.5994)
  line L113 (-111.1055, -24.5994) -> (-115.106, -24.5994)
  line L114 (-115.106, -24.5994) -> (-115.106, -10.5999)
  line L115 (-115.106, -10.5999) -> (-111.1055, -10.5999)
  line L116 (-111.1055, -10.5999) -> (-111.1055, -9.5999)
  line L117 (-111.1055, -9.5999) -> (-105.1055, -9.5999)
  line L118 (-105.1055, -9.5999) -> (-105.1055, -10.5999)
  line L119 (-105.1055, -10.5999) -> (-101.105, -10.5999)
  line L120 (-101.105, -10.5999) -> (-101.105, -24.5994)
  line L121 (-101.105, -24.5994) -> (-105.1055, -24.5994)
  line L122 (-105.1055, -24.5994) -> (-105.1055, -25.5994)
  line L123 (-105.1055, -25.5994) -> (-111.1055, -25.5994)
  line L124 (-14.6183, -43.6492) -> (-14.6183, -44.6492)
  line L125 (-14.6183, -44.6492) -> (-20.6183, -44.6492)
  line L126 (-20.6183, -44.6492) -> (-20.6183, -43.6492)
  line L127 (-20.6183, -43.6492) -> (-24.6187, -43.6492)
  line L128 (-24.6187, -43.6492) -> (-24.6187, -29.6499)
  line L129 (-24.6187, -29.6499) -> (-20.6183, -29.6499)
  line L130 (-20.6183, -29.6499) -> (-20.6183, -28.6499)
  line L131 (-20.6183, -28.6499) -> (-14.6183, -28.6499)
  line L132 (-14.6183, -28.6499) -> (-14.6183, -29.6499)
  line L133 (-14.6183, -29.6499) -> (-10.6178, -29.6499)
  line L134 (-10.6178, -29.6499) -> (-10.6178, -43.6492)
  line L135 (-10.6178, -43.6492) -> (-14.6183, -43.6492)
  line L136 (-130.1555, -25.5994) -> (-130.1555, -24.5994)
  line L137 (-130.1555, -24.5994) -> (-134.156, -24.5994)
  line L138 (-134.156, -24.5994) -> (-134.156, -10.5999)
  line L139 (-134.156, -10.5999) -> (-130.1555, -10.5999)
  line L140 (-130.1555, -10.5999) -> (-130.1555, -9.5999)
  line L141 (-130.1555, -9.5999) -> (-124.1555, -9.5999)
  line L142 (-124.1555, -9.5999) -> (-124.1555, -10.5999)
  line L143 (-124.1555, -10.5999) -> (-120.155, -10.5999)
  line L144 (-120.155, -10.5999) -> (-120.155, -24.5994)
  line L145 (-120.155, -24.5994) -> (-124.1555, -24.5994)
  line L146 (-124.1555, -24.5994) -> (-124.1555, -25.5994)
  line L147 (-124.1555, -25.5994) -> (-130.1555, -25.5994)
  line L148 (-133.6805, -28.6499) -> (-133.6805, -29.6499)
  line L149 (-133.6805, -29.6499) -> (-129.68, -29.6499)
  line L150 (-129.68, -29.6499) -> (-129.68, -43.6492)
  line L151 (-129.68, -43.6492) -> (-133.6805, -43.6492)
  line L152 (-133.6805, -43.6492) -> (-133.6805, -44.6492)
  line L153 (-133.6805, -44.6492) -> (-139.6805, -44.6492)
  line L154 (-139.6805, -44.6492) -> (-139.6805, -43.6492)
  line L155 (-139.6805, -43.6492) -> (-143.681, -43.6492)
  line L156 (-143.681, -43.6492) -> (-143.681, -29.6499)
  line L157 (-143.681, -29.6499) -> (-139.6805, -29.6499)
  line L158 (-139.6805, -29.6499) -> (-139.6805, -28.6499)
  line L159 (-139.6805, -28.6499) -> (-133.6805, -28.6499)
  line L160 (-49.1926, -25.5994) -> (-49.1926, -24.5994)
  line L161 (-49.1926, -24.5994) -> (-53.1922, -24.5994)
  line L162 (-53.1922, -24.5994) -> (-53.1922, -10.5999)
  line L163 (-53.1922, -10.5999) -> (-49.1926, -10.5999)
  line L164 (-49.1926, -10.5999) -> (-49.1926, -9.5999)
  line L165 (-49.1926, -9.5999) -> (-43.1926, -9.5999)
  line L166 (-43.1926, -9.5999) -> (-43.1926, -10.5999)
  line L167 (-43.1926, -10.5999) -> (-39.1929, -10.5999)
  line L168 (-39.1929, -10.5999) -> (-39.1929, -24.5994)
  line L169 (-39.1929, -24.5994) -> (-43.1926, -24.5994)
  line L170 (-43.1926, -24.5994) -> (-43.1926, -25.5994)
  line L171 (-43.1926, -25.5994) -> (-49.1926, -25.5994)
  line L172 (-39.6689, -44.6492) -> (-39.6689, -43.6492)
  line L173 (-39.6689, -43.6492) -> (-43.6686, -43.6492)
  line L174 (-43.6686, -43.6492) -> (-43.6686, -29.6499)
  line L175 (-43.6686, -29.6499) -> (-39.6689, -29.6499)
  line L176 (-39.6689, -29.6499) -> (-39.6689, -28.6499)
  line L177 (-39.6689, -28.6499) -> (-33.6689, -28.6499)
  line L178 (-33.6689, -28.6499) -> (-33.6689, -29.6499)
  line L179 (-33.6689, -29.6499) -> (-29.6692, -29.6499)
  line L180 (-29.6692, -29.6499) -> (-29.6692, -43.6492)
  line L181 (-29.6692, -43.6492) -> (-33.6689, -43.6492)
  line L182 (-33.6689, -43.6492) -> (-33.6689, -44.6492)
  line L183 (-33.6689, -44.6492) -> (-39.6689, -44.6492)
  line L184 (-105.581, -65.2253) -> (-148.73, -65.2253) construction
  circle A0 centre (-127.1555, -65.2253) radius 4.65
  line L185 (-46.1926, -25.5994) -> (-46.1926, -65.2253) construction
  line L186 (-46.1926, -65.2253) -> (-67.7693, -65.2253) construction
  circle A1 centre (-46.1926, -65.2253) radius 4.65
  circle A2 centre (-5.0937, -77.7497) radius 1.75
  circle A3 centre (-5.0937, -5.0744) radius 1.75
  circle A4 centre (-168.257, -5.0744) radius 1.75
  circle A5 centre (-168.257, -77.7497) radius 1.75
  dimension "d65" = 9.3
  dimension "d66" = 9.3
  dimension "d67" = 3.5
  dimension "d68" = 3.5
  dimension "d69" = 3.5
  dimension "d70" = 3.5
  dimension "d71" = 5
  dimension "d72" = 5
  dimension "d73" = 5
  dimension "d74" = 5
  dimension "d75" = 5
  dimension "d76" = 5
  dimension "d77" = 5
  dimension "d78" = 5
  constraint midpoint L14 L184.start
  constraint midpoint L26 L184.end
  constraint midpoint L184 A0.centre
  constraint midpoint L171 L185.start
  constraint perpendicular L171 L185
  constraint midpoint L62 L186.end
  constraint perpendicular L62 L186
  constraint coincident L185.end L186.start
  measures "d65" diameter of A0
  measures "d66" diameter of A1
  measures "d67" diameter of A2
  measures "d68" diameter of A3
  measures "d69" diameter of A4
  measures "d70" diameter of A5
  measures "d71" distance of L3 A5.centre
  measures "d72" distance of L0 A5.centre
  measures "d73" distance of L2 A4.centre
  measures "d74" distance of L3 A4.centre
  measures "d75" distance of L1 A3.centre
  measures "d76" distance of L2 A3.centre
  measures "d77" distance of L1 A2.centre
  measures "d78" distance of L0 A2.centre
extrude "Extrude3" cut sketch "Sketch3" against normal blind 3 contours A0 | A1 | A2 | A3 | A4 | A5
sketch "Sketch2 (2)" plane through (0, 0, 3) normal (0, 0, 1) x (-1, 0, 0)
  circle A0 centre (-5.0937, -5.0744) radius 1.75
  circle A1 centre (-127.1555, -65.2253) radius 4.65
  circle A2 centre (-5.0937, -77.7497) radius 1.75
  circle A3 centre (-168.257, -5.0744) radius 1.75
  circle A4 centre (-168.257, -77.7497) radius 1.75
  circle A5 centre (-46.1926, -65.2253) radius 4.65
  line L0 (-173.257, -82.7497) -> (-0.0937, -82.7497)
  line L1 (-0.0937, -82.7497) -> (-0.0937, -0.0744)
  line L2 (-0.0937, -0.0744) -> (-173.257, -0.0744)
  line L3 (-173.257, -0.0744) -> (-173.257, -82.7497)
  line L4 (-152.7305, -72.2256) -> (-152.7305, -73.2256)
  line L5 (-152.7305, -73.2256) -> (-158.7305, -73.2256)
  line L6 (-158.7305, -73.2256) -> (-158.7305, -72.2256)
  line L7 (-158.7305, -72.2256) -> (-162.731, -72.2256)
  line L8 (-162.731, -72.2256) -> (-162.731, -58.2249)
  line L9 (-162.731, -58.2249) -> (-158.7305, -58.2249)
  line L10 (-158.7305, -58.2249) -> (-158.7305, -57.2249)
  line L11 (-158.7305, -57.2249) -> (-152.7305, -57.2249)
  line L12 (-152.7305, -57.2249) -> (-152.7305, -58.2249)
  line L13 (-152.7305, -58.2249) -> (-148.73, -58.2249)
  line L14 (-148.73, -58.2249) -> (-148.73, -72.2256)
  line L15 (-148.73, -72.2256) -> (-152.7305, -72.2256)
  line L16 (-101.5807, -58.2249) -> (-101.5807, -57.2249)
  line L17 (-101.5807, -57.2249) -> (-95.5807, -57.2249)
  line L18 (-95.5807, -57.2249) -> (-95.5807, -58.2249)
  line L19 (-95.5807, -58.2249) -> (-91.5804, -58.2249)
  line L20 (-91.5804, -58.2249) -> (-91.5804, -72.2256)
  line L21 (-91.5804, -72.2256) -> (-95.5807, -72.2256)
  line L22 (-95.5807, -72.2256) -> (-95.5807, -73.2256)
  line L23 (-95.5807, -73.2256) -> (-101.5807, -73.2256)
  line L24 (-101.5807, -73.2256) -> (-101.5807, -72.2256)
  line L25 (-101.5807, -72.2256) -> (-105.581, -72.2256)
  line L26 (-105.581, -72.2256) -> (-105.581, -58.2249)
  line L27 (-105.581, -58.2249) -> (-101.5807, -58.2249)
  line L28 (-58.7189, -44.6492) -> (-58.7189, -43.6492)
  line L29 (-58.7189, -43.6492) -> (-62.7186, -43.6492)
  line L30 (-62.7186, -43.6492) -> (-62.7186, -29.6499)
  line L31 (-62.7186, -29.6499) -> (-58.719, -29.6499)
  line L32 (-58.719, -29.6499) -> (-58.719, -28.6499)
  line L33 (-58.719, -28.6499) -> (-52.7189, -28.6499)
  line L34 (-52.7189, -28.6499) -> (-52.7189, -29.6499)
  line L35 (-52.7189, -29.6499) -> (-48.7193, -29.6499)
  line L36 (-48.7193, -29.6499) -> (-48.7193, -43.6492)
  line L37 (-48.7193, -43.6492) -> (-52.7189, -43.6492)
  line L38 (-52.7189, -43.6492) -> (-52.7189, -44.6492)
  line L39 (-52.7189, -44.6492) -> (-58.7189, -44.6492)
  line L40 (-24.1433, -24.5994) -> (-24.1433, -25.5994)
  line L41 (-24.1433, -25.5994) -> (-30.1433, -25.5994)
  line L42 (-30.1433, -25.5994) -> (-30.1433, -24.5994)
  line L43 (-30.1433, -24.5994) -> (-34.1437, -24.5994)
  line L44 (-34.1437, -24.5994) -> (-34.1437, -10.5999)
  line L45 (-34.1437, -10.5999) -> (-30.1433, -10.5999)
  line L46 (-30.1433, -10.5999) -> (-30.1433, -9.5999)
  line L47 (-30.1433, -9.5999) -> (-24.1433, -9.5999)
  line L48 (-24.1433, -9.5999) -> (-24.1433, -10.5999)
  line L49 (-24.1433, -10.5999) -> (-20.1428, -10.5999)
  line L50 (-20.1428, -10.5999) -> (-20.1428, -24.5994)
  line L51 (-20.1428, -24.5994) -> (-24.1433, -24.5994)
  line L52 (-71.769, -72.2256) -> (-71.769, -73.2256)
  line L53 (-71.769, -73.2256) -> (-77.769, -73.2256)
  line L54 (-77.769, -73.2256) -> (-77.769, -72.2256)
  line L55 (-77.769, -72.2256) -> (-81.7686, -72.2256)
  line L56 (-81.7686, -72.2256) -> (-81.7686, -58.2249)
  line L57 (-81.7686, -58.2249) -> (-77.769, -58.2249)
  line L58 (-77.769, -58.2249) -> (-77.769, -57.2249)
  line L59 (-77.769, -57.2249) -> (-71.769, -57.2249)
  line L60 (-71.769, -57.2249) -> (-71.769, -58.2249)
  line L61 (-71.769, -58.2249) -> (-67.7693, -58.2249)
  line L62 (-67.7693, -58.2249) -> (-67.7693, -72.2256)
  line L63 (-67.7693, -72.2256) -> (-71.769, -72.2256)
  line L64 (-158.7305, -44.6492) -> (-158.7305, -43.6492)
  line L65 (-158.7305, -43.6492) -> (-162.731, -43.6492)
  line L66 (-162.731, -43.6492) -> (-162.731, -29.6499)
  line L67 (-162.731, -29.6499) -> (-158.7305, -29.6499)
  line L68 (-158.7305, -29.6499) -> (-158.7305, -28.6499)
  line L69 (-158.7305, -28.6499) -> (-152.7305, -28.6499)
  line L70 (-152.7305, -28.6499) -> (-152.7305, -29.6499)
  line L71 (-152.7305, -29.6499) -> (-148.73, -29.6499)
  line L72 (-148.73, -29.6499) -> (-148.73, -43.6492)
  line L73 (-148.73, -43.6492) -> (-152.7305, -43.6492)
  line L74 (-152.7305, -43.6492) -> (-152.7305, -44.6492)
  line L75 (-152.7305, -44.6492) -> (-158.7305, -44.6492)
  line L76 (-149.2055, -25.5994) -> (-149.2055, -24.5994)
  line L77 (-149.2055, -24.5994) -> (-153.206, -24.5994)
  line L78 (-153.206, -24.5994) -> (-153.206, -10.5999)
  line L79 (-153.206, -10.5999) -> (-149.2055, -10.5999)
  line L80 (-149.2055, -10.5999) -> (-149.2055, -9.5999)
  line L81 (-149.2055, -9.5999) -> (-143.2055, -9.5999)
  line L82 (-143.2055, -9.5999) -> (-143.2055, -10.5999)
  line L83 (-143.2055, -10.5999) -> (-139.205, -10.5999)
  line L84 (-139.205, -10.5999) -> (-139.205, -24.5994)
  line L85 (-139.205, -24.5994) -> (-143.2055, -24.5994)
  line L86 (-143.2055, -24.5994) -> (-143.2055, -25.5994)
  line L87 (-143.2055, -25.5994) -> (-149.2055, -25.5994)
  line L88 (-62.2426, -9.5999) -> (-62.2426, -10.5999)
  line L89 (-62.2426, -10.5999) -> (-58.2429, -10.5999)
  line L90 (-58.2429, -10.5999) -> (-58.2429, -24.5994)
  line L91 (-58.2429, -24.5994) -> (-62.2426, -24.5994)
  line L92 (-62.2426, -24.5994) -> (-62.2426, -25.5994)
  line L93 (-62.2426, -25.5994) -> (-68.2425, -25.5994)
  line L94 (-68.2425, -25.5994) -> (-68.2425, -24.5994)
  line L95 (-68.2425, -24.5994) -> (-72.2422, -24.5994)
  line L96 (-72.2422, -24.5994) -> (-72.2422, -10.5999)
  line L97 (-72.2422, -10.5999) -> (-68.2426, -10.5999)
  line L98 (-68.2426, -10.5999) -> (-68.2426, -9.5999)
  line L99 (-68.2426, -9.5999) -> (-62.2426, -9.5999)
  line L100 (-114.6305, -28.6499) -> (-114.6305, -29.6499)
  line L101 (-114.6305, -29.6499) -> (-110.63, -29.6499)
  line L102 (-110.63, -29.6499) -> (-110.63, -43.6492)
  line L103 (-110.63, -43.6492) -> (-114.6305, -43.6492)
  line L104 (-114.6305, -43.6492) -> (-114.6305, -44.6492)
  line L105 (-114.6305, -44.6492) -> (-120.6305, -44.6492)
  line L106 (-120.6305, -44.6492) -> (-120.6305, -43.6492)
  line L107 (-120.6305, -43.6492) -> (-124.631, -43.6492)
  line L108 (-124.631, -43.6492) -> (-124.631, -29.6499)
  line L109 (-124.631, -29.6499) -> (-120.6305, -29.6499)
  line L110 (-120.6305, -29.6499) -> (-120.6305, -28.6499)
  line L111 (-120.6305, -28.6499) -> (-114.6305, -28.6499)
  line L112 (-111.1055, -25.5994) -> (-111.1055, -24.5994)
  line L113 (-111.1055, -24.5994) -> (-115.106, -24.5994)
  line L114 (-115.106, -24.5994) -> (-115.106, -10.5999)
  line L115 (-115.106, -10.5999) -> (-111.1055, -10.5999)
  line L116 (-111.1055, -10.5999) -> (-111.1055, -9.5999)
  line L117 (-111.1055, -9.5999) -> (-105.1055, -9.5999)
  line L118 (-105.1055, -9.5999) -> (-105.1055, -10.5999)
  line L119 (-105.1055, -10.5999) -> (-101.105, -10.5999)
  line L120 (-101.105, -10.5999) -> (-101.105, -24.5994)
  line L121 (-101.105, -24.5994) -> (-105.1055, -24.5994)
  line L122 (-105.1055, -24.5994) -> (-105.1055, -25.5994)
  line L123 (-105.1055, -25.5994) -> (-111.1055, -25.5994)
  line L124 (-14.6183, -43.6492) -> (-14.6183, -44.6492)
  line L125 (-14.6183, -44.6492) -> (-20.6183, -44.6492)
  line L126 (-20.6183, -44.6492) -> (-20.6183, -43.6492)
  line L127 (-20.6183, -43.6492) -> (-24.6187, -43.6492)
  line L128 (-24.6187, -43.6492) -> (-24.6187, -29.6499)
  line L129 (-24.6187, -29.6499) -> (-20.6183, -29.6499)
  line L130 (-20.6183, -29.6499) -> (-20.6183, -28.6499)
  line L131 (-20.6183, -28.6499) -> (-14.6183, -28.6499)
  line L132 (-14.6183, -28.6499) -> (-14.6183, -29.6499)
  line L133 (-14.6183, -29.6499) -> (-10.6178, -29.6499)
  line L134 (-10.6178, -29.6499) -> (-10.6178, -43.6492)
  line L135 (-10.6178, -43.6492) -> (-14.6183, -43.6492)
  line L136 (-130.1555, -25.5994) -> (-130.1555, -24.5994)
  line L137 (-130.1555, -24.5994) -> (-134.156, -24.5994)
  line L138 (-134.156, -24.5994) -> (-134.156, -10.5999)
  line L139 (-134.156, -10.5999) -> (-130.1555, -10.5999)
  line L140 (-130.1555, -10.5999) -> (-130.1555, -9.5999)
  line L141 (-130.1555, -9.5999) -> (-124.1555, -9.5999)
  line L142 (-124.1555, -9.5999) -> (-124.1555, -10.5999)
  line L143 (-124.1555, -10.5999) -> (-120.155, -10.5999)
  line L144 (-120.155, -10.5999) -> (-120.155, -24.5994)
  line L145 (-120.155, -24.5994) -> (-124.1555, -24.5994)
  line L146 (-124.1555, -24.5994) -> (-124.1555, -25.5994)
  line L147 (-124.1555, -25.5994) -> (-130.1555, -25.5994)
  line L148 (-133.6805, -28.6499) -> (-133.6805, -29.6499)
  line L149 (-133.6805, -29.6499) -> (-129.68, -29.6499)
  line L150 (-129.68, -29.6499) -> (-129.68, -43.6492)
  line L151 (-129.68, -43.6492) -> (-133.6805, -43.6492)
  line L152 (-133.6805, -43.6492) -> (-133.6805, -44.6492)
  line L153 (-133.6805, -44.6492) -> (-139.6805, -44.6492)
  line L154 (-139.6805, -44.6492) -> (-139.6805, -43.6492)
  line L155 (-139.6805, -43.6492) -> (-143.681, -43.6492)
  line L156 (-143.681, -43.6492) -> (-143.681, -29.6499)
  line L157 (-143.681, -29.6499) -> (-139.6805, -29.6499)
  line L158 (-139.6805, -29.6499) -> (-139.6805, -28.6499)
  line L159 (-139.6805, -28.6499) -> (-133.6805, -28.6499)
  line L160 (-49.1926, -25.5994) -> (-49.1926, -24.5994)
  line L161 (-49.1926, -24.5994) -> (-53.1922, -24.5994)
  line L162 (-53.1922, -24.5994) -> (-53.1922, -10.5999)
  line L163 (-53.1922, -10.5999) -> (-49.1926, -10.5999)
  line L164 (-49.1926, -10.5999) -> (-49.1926, -9.5999)
  line L165 (-49.1926, -9.5999) -> (-43.1926, -9.5999)
  line L166 (-43.1926, -9.5999) -> (-43.1926, -10.5999)
  line L167 (-43.1926, -10.5999) -> (-39.1929, -10.5999)
  line L168 (-39.1929, -10.5999) -> (-39.1929, -24.5994)
  line L169 (-39.1929, -24.5994) -> (-43.1926, -24.5994)
  line L170 (-43.1926, -24.5994) -> (-43.1926, -25.5994)
  line L171 (-43.1926, -25.5994) -> (-49.1926, -25.5994)
  line L172 (-39.6689, -44.6492) -> (-39.6689, -43.6492)
  line L173 (-39.6689, -43.6492) -> (-43.6686, -43.6492)
  line L174 (-43.6686, -43.6492) -> (-43.6686, -29.6499)
  line L175 (-43.6686, -29.6499) -> (-39.6689, -29.6499)
  line L176 (-39.6689, -29.6499) -> (-39.6689, -28.6499)
  line L177 (-39.6689, -28.6499) -> (-33.6689, -28.6499)
  line L178 (-33.6689, -28.6499) -> (-33.6689, -29.6499)
  line L179 (-33.6689, -29.6499) -> (-29.6692, -29.6499)
  line L180 (-29.6692, -29.6499) -> (-29.6692, -43.6492)
  line L181 (-29.6692, -43.6492) -> (-33.6689, -43.6492)
  line L182 (-33.6689, -43.6492) -> (-33.6689, -44.6492)
  line L183 (-33.6689, -44.6492) -> (-39.6689, -44.6492)
  line L184 (-46.1926, -65.2253) -> (-55.1926, -65.2253) construction
  circle A6 centre (-55.1926, -65.2253) radius 1.75
  line L185 (-127.1555, -65.2253) -> (-118.1555, -65.2253) construction
  circle A7 centre (-118.1555, -65.2253) radius 1.75
  dimension "d85" = 9
  dimension "d86" = 3.5
  dimension "d87" = 9
  dimension "d88" = 3.5
  constraint coincident A5.centre L184.start
  constraint horizontal L184
  constraint coincident L184.end A6.centre
  constraint coincident A1.centre L185.start
  constraint horizontal L185
  constraint coincident L185.end A7.centre
  measures "d85" distance of A5.centre L184.end
  measures "d86" diameter of A6
  measures "d87" distance of A1.centre L185.end
  measures "d88" diameter of A7
extrude "Extrude1'" cut sketch "Sketch2 (2)" against normal blind 2 contours A6 | A7